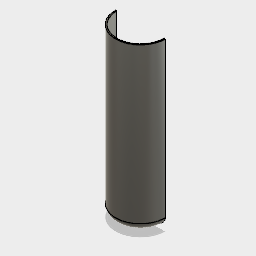
PRV_under v1 (Autodesk Fusion 360 design; units mm, degrees)
Autodesk Fusion 360 part; units mm, degrees
sketch "スケッチ1" plane through (0, 0, 0) normal (0, 0, 1) x (1, 0, 0)
  line L0 (2750, 1300) -> (2750, 18400)
  line L1 (0, 0) -> (0, 140)
  ellipse E0 centre (0, 1300) end of major axis (0, 0) minor radius 2750 (0, 0) -> (2750, 1300) ccw
  line L2 (2750, 1300) -> (2610, 1300)
  ellipse E1 centre (0, 1300) end of major axis (0, 140) minor radius 2610 (0, 140) -> (2610, 1300) ccw
  line L3 (2610, 1300) -> (2610, 18400)
  line L4 (2610, 18400) -> (2750, 18400)
  dimension "d3" = 140
  dimension "d7" = 140
  dimension "d8" = 17100
  measures "d3" distance of L1.start L1.end
  measures "d7" distance of L0.start L2.end
  measures "d8" distance of L2.end L3.end
revolve "回転1" add sketch "スケッチ1" angle 180 about axis through (0, 1.75, 0) along (0, -1, 0)
equation "d8 = 1.710E+04 mm"
